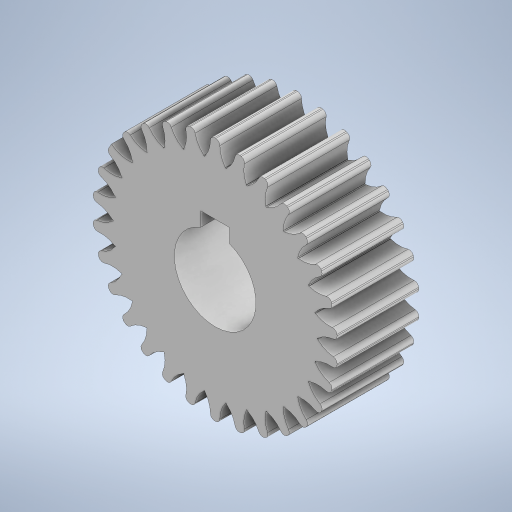
# Autodesk Inventor part: ENGRANE
Saved by Autodesk Inventor 2024 (Build 280153000, 153)
## iProperties
Created: 2024-03-04
Part Number: ENGRANE
Material: Generic
Document SubType Name: Modeling
Designer: augus
Density: 1 g/cm^3
Appearance: Default
Author: augus
Autodesk Inventor part; units mm, degrees
ref_plane "YZ Plane" through (0, 0, 0) normal (1, 0, 0) x (0, 1, 0)
ref_plane "XZ Plane" through (0, 0, 0) normal (0, 1, 0) x (-1, 0, 0)
ref_plane "XY Plane" through (0, 0, 0) normal (0, 0, 1) x (1, 0, 0)
sketch "Sketch1" plane through (0, 0, 0) normal (0, 0, 1) x (1, 0, 0)
  circle A0 centre (0, 0) radius 25
  line L0 (-1.25, 30) -> (1.25, 30)
  line L1 (2.5, 25) -> (2.5, 20)
  line L2 (2.5, 20) -> (-2.5, 20)
  line L3 (-2.5, 20) -> (-2.5, 25)
  line L4 (-1.2964, 27.5929) -> (2.5, 20) construction
  line L5 (1.2964, 27.5929) -> (-2.5, 20) construction
  arc A1 (-2.5, 25) -> (-1.25, 30) centre (-7.5449, 28.9175) ccw
  arc A2 (1.25, 30) -> (2.5, 25) centre (7.5449, 28.9175) ccw
  line L6 (-7.46, 29.0845) -> (-5.0147, 29.6043)
  arc A3 (-5.0147, 29.6043) -> (-2.7524, 24.9735) centre (1.3677, 29.8542) ccw
  arc A4 (-7.6432, 23.9339) -> (-7.46, 29.0845) centre (-13.3923, 26.7169) ccw
  line L7 (-6.6036, 19.0432) -> (-7.6432, 23.9339)
  line L8 (-2.7524, 24.9735) -> (-1.7129, 20.0827)
  line L9 (-1.7129, 20.0827) -> (-6.6036, 19.0432)
  line L10 (-13.344, 26.8979) -> (-11.0602, 27.9148)
  arc A5 (-11.0602, 27.9148) -> (-7.8846, 23.8555) centre (-4.8692, 29.4862) ccw
  arc A6 (-12.4523, 21.8218) -> (-13.344, 26.8979) centre (-18.6544, 23.3486) ccw
  line L11 (-10.4186, 17.2541) -> (-12.4523, 21.8218)
  line L12 (-7.8846, 23.8555) -> (-5.8509, 19.2878)
  line L13 (-5.8509, 19.2878) -> (-10.4186, 17.2541)
  line L14 (-18.6448, 23.5358) -> (-16.6223, 25.0052)
  arc A7 (-16.6223, 25.0052) -> (-12.6721, 21.6949) centre (-10.8933, 27.8295) ccw
  arc A8 (-16.7172, 18.756) -> (-18.6448, 23.5358) centre (-23.1012, 18.96) ccw
  line L15 (-13.7782, 14.7109) -> (-16.7172, 18.756)
  line L16 (-12.6721, 21.6949) -> (-9.7332, 17.6498)
  line L17 (-9.7332, 17.6498) -> (-13.7782, 14.7109)
  line L18 (-23.1308, 19.145) -> (-21.4579, 21.0028)
  arc A9 (-21.4579, 21.0028) -> (-16.9058, 18.5861) centre (-16.4414, 24.9565) ccw
  arc A10 (-20.2514, 14.8704) -> (-23.1308, 19.145) centre (-26.5384, 13.7426) ccw
  line L19 (-16.5357, 11.5248) -> (-20.2514, 14.8704)
  line L20 (-16.9058, 18.5861) -> (-13.1901, 15.2405)
  line L21 (-13.1901, 15.2405) -> (-16.5357, 11.5248)
  line L22 (-26.6058, 13.9175) -> (-25.3558, 16.0825)
  arc A11 (-25.3558, 16.0825) -> (-20.4006, 14.6651) centre (-21.2708, 20.9928) ccw
  arc A12 (-22.9006, 10.3349) -> (-26.6058, 13.9175) centre (-28.8157, 7.9247) ccw
  line L23 (-18.5705, 7.8349) -> (-22.9006, 10.3349)
  line L24 (-20.4006, 14.6651) -> (-16.0705, 12.1651)
  line L25 (-16.0705, 12.1651) -> (-18.5705, 7.8349)
  line L26 (-28.918, 8.0817) -> (-28.1454, 10.4593)
  arc A13 (-28.1454, 10.4593) -> (-23.0039, 10.1031) centre (-25.1707, 16.1116) ccw
  arc A14 (-24.549, 5.3478) -> (-28.918, 8.0817) centre (-29.8336, 1.7604) ccw
  line L27 (-19.7937, 3.8027) -> (-24.549, 5.3478)
  line L28 (-23.0039, 10.1031) -> (-18.2486, 8.558)
  line L29 (-18.2486, 8.558) -> (-19.7937, 3.8027)
  line L30 (-29.9663, 1.8927) -> (-29.705, 4.379)
  arc A15 (-29.705, 4.379) -> (-24.6017, 5.0995) centre (-27.9704, 10.5262) ccw
  arc A16 (-25.1244, 0.1269) -> (-29.9663, 1.8927) centre (-29.5477, -4.4808) ccw
  line L31 (-20.1518, -0.3957) -> (-25.1244, 0.1269)
  line L32 (-24.6017, 5.0995) -> (-19.6291, 4.5769)
  line L33 (-19.6291, 4.5769) -> (-20.1518, -0.3957)
  line L34 (-29.705, -4.379) -> (-29.9663, -1.8927)
  arc A17 (-29.9663, -1.8927) -> (-25.1244, -0.1269) centre (-29.5477, 4.4808) ccw
  arc A18 (-24.6017, -5.0995) -> (-29.705, -4.379) centre (-27.9704, -10.5262) ccw
  line L35 (-19.6291, -4.5769) -> (-24.6017, -5.0995)
  line L36 (-25.1244, -0.1269) -> (-20.1518, 0.3957)
  line L37 (-20.1518, 0.3957) -> (-19.6291, -4.5769)
  line L38 (-28.1454, -10.4593) -> (-28.918, -8.0817)
  arc A19 (-28.918, -8.0817) -> (-24.549, -5.3478) centre (-29.8336, -1.7604) ccw
  arc A20 (-23.0039, -10.1031) -> (-28.1454, -10.4593) centre (-25.1707, -16.1116) ccw
  line L39 (-18.2486, -8.558) -> (-23.0039, -10.1031)
  line L40 (-24.549, -5.3478) -> (-19.7937, -3.8027)
  line L41 (-19.7937, -3.8027) -> (-18.2486, -8.558)
  line L42 (-25.3558, -16.0825) -> (-26.6058, -13.9175)
  arc A21 (-26.6058, -13.9175) -> (-22.9006, -10.3349) centre (-28.8157, -7.9247) ccw
  arc A22 (-20.4006, -14.6651) -> (-25.3558, -16.0825) centre (-21.2708, -20.9928) ccw
  line L43 (-16.0705, -12.1651) -> (-20.4006, -14.6651)
  line L44 (-22.9006, -10.3349) -> (-18.5705, -7.8349)
  line L45 (-18.5705, -7.8349) -> (-16.0705, -12.1651)
  line L46 (-21.4579, -21.0028) -> (-23.1308, -19.145)
  arc A23 (-23.1308, -19.145) -> (-20.2514, -14.8704) centre (-26.5384, -13.7426) ccw
  arc A24 (-16.9058, -18.5861) -> (-21.4579, -21.0028) centre (-16.4414, -24.9565) ccw
  line L47 (-13.1901, -15.2405) -> (-16.9058, -18.5861)
  line L48 (-20.2514, -14.8704) -> (-16.5357, -11.5248)
  line L49 (-16.5357, -11.5248) -> (-13.1901, -15.2405)
  line L50 (-16.6223, -25.0052) -> (-18.6448, -23.5358)
  arc A25 (-18.6448, -23.5358) -> (-16.7172, -18.756) centre (-23.1012, -18.96) ccw
  arc A26 (-12.6721, -21.6949) -> (-16.6223, -25.0052) centre (-10.8933, -27.8295) ccw
  line L51 (-9.7332, -17.6498) -> (-12.6721, -21.6949)
  line L52 (-16.7172, -18.756) -> (-13.7782, -14.7109)
  line L53 (-13.7782, -14.7109) -> (-9.7332, -17.6498)
  line L54 (-11.0602, -27.9148) -> (-13.344, -26.8979)
  arc A27 (-13.344, -26.8979) -> (-12.4523, -21.8218) centre (-18.6544, -23.3486) ccw
  arc A28 (-7.8846, -23.8555) -> (-11.0602, -27.9148) centre (-4.8692, -29.4862) ccw
  line L55 (-5.8509, -19.2878) -> (-7.8846, -23.8555)
  line L56 (-12.4523, -21.8218) -> (-10.4186, -17.2541)
  line L57 (-10.4186, -17.2541) -> (-5.8509, -19.2878)
  line L58 (-5.0147, -29.6043) -> (-7.46, -29.0845)
  arc A29 (-7.46, -29.0845) -> (-7.6432, -23.9339) centre (-13.3923, -26.7169) ccw
  arc A30 (-2.7524, -24.9735) -> (-5.0147, -29.6043) centre (1.3677, -29.8542) ccw
  line L59 (-1.7129, -20.0827) -> (-2.7524, -24.9735)
  line L60 (-7.6432, -23.9339) -> (-6.6036, -19.0432)
  line L61 (-6.6036, -19.0432) -> (-1.7129, -20.0827)
  line L62 (1.25, -30) -> (-1.25, -30)
  arc A31 (-1.25, -30) -> (-2.5, -25) centre (-7.5449, -28.9175) ccw
  arc A32 (2.5, -25) -> (1.25, -30) centre (7.5449, -28.9175) ccw
  line L63 (2.5, -20) -> (2.5, -25)
  line L64 (-2.5, -25) -> (-2.5, -20)
  line L65 (-2.5, -20) -> (2.5, -20)
  line L66 (7.46, -29.0845) -> (5.0147, -29.6043)
  arc A33 (5.0147, -29.6043) -> (2.7524, -24.9735) centre (-1.3677, -29.8542) ccw
  arc A34 (7.6432, -23.9339) -> (7.46, -29.0845) centre (13.3923, -26.7169) ccw
  line L67 (6.6036, -19.0432) -> (7.6432, -23.9339)
  line L68 (2.7524, -24.9735) -> (1.7129, -20.0827)
  line L69 (1.7129, -20.0827) -> (6.6036, -19.0432)
  line L70 (13.344, -26.8979) -> (11.0602, -27.9148)
  arc A35 (11.0602, -27.9148) -> (7.8846, -23.8555) centre (4.8692, -29.4862) ccw
  arc A36 (12.4523, -21.8218) -> (13.344, -26.8979) centre (18.6544, -23.3486) ccw
  line L71 (10.4186, -17.2541) -> (12.4523, -21.8218)
  line L72 (7.8846, -23.8555) -> (5.8509, -19.2878)
  line L73 (5.8509, -19.2878) -> (10.4186, -17.2541)
  line L74 (18.6448, -23.5358) -> (16.6223, -25.0052)
  arc A37 (16.6223, -25.0052) -> (12.6721, -21.6949) centre (10.8933, -27.8295) ccw
  arc A38 (16.7172, -18.756) -> (18.6448, -23.5358) centre (23.1012, -18.96) ccw
  line L75 (13.7782, -14.7109) -> (16.7172, -18.756)
  line L76 (12.6721, -21.6949) -> (9.7332, -17.6498)
  line L77 (9.7332, -17.6498) -> (13.7782, -14.7109)
  line L78 (23.1308, -19.145) -> (21.4579, -21.0028)
  arc A39 (21.4579, -21.0028) -> (16.9058, -18.5861) centre (16.4414, -24.9565) ccw
  arc A40 (20.2514, -14.8704) -> (23.1308, -19.145) centre (26.5384, -13.7426) ccw
  line L79 (16.5357, -11.5248) -> (20.2514, -14.8704)
  line L80 (16.9058, -18.5861) -> (13.1901, -15.2405)
  line L81 (13.1901, -15.2405) -> (16.5357, -11.5248)
  line L82 (26.6058, -13.9175) -> (25.3558, -16.0825)
  arc A41 (25.3558, -16.0825) -> (20.4006, -14.6651) centre (21.2708, -20.9928) ccw
  arc A42 (22.9006, -10.3349) -> (26.6058, -13.9175) centre (28.8157, -7.9247) ccw
  line L83 (18.5705, -7.8349) -> (22.9006, -10.3349)
  line L84 (20.4006, -14.6651) -> (16.0705, -12.1651)
  line L85 (16.0705, -12.1651) -> (18.5705, -7.8349)
  line L86 (28.918, -8.0817) -> (28.1454, -10.4593)
  arc A43 (28.1454, -10.4593) -> (23.0039, -10.1031) centre (25.1707, -16.1116) ccw
  arc A44 (24.549, -5.3478) -> (28.918, -8.0817) centre (29.8336, -1.7604) ccw
  line L87 (19.7937, -3.8027) -> (24.549, -5.3478)
  line L88 (23.0039, -10.1031) -> (18.2486, -8.558)
  line L89 (18.2486, -8.558) -> (19.7937, -3.8027)
  line L90 (29.9663, -1.8927) -> (29.705, -4.379)
  arc A45 (29.705, -4.379) -> (24.6017, -5.0995) centre (27.9704, -10.5262) ccw
  arc A46 (25.1244, -0.1269) -> (29.9663, -1.8927) centre (29.5477, 4.4808) ccw
  line L91 (20.1518, 0.3957) -> (25.1244, -0.1269)
  line L92 (24.6017, -5.0995) -> (19.6291, -4.5769)
  line L93 (19.6291, -4.5769) -> (20.1518, 0.3957)
  line L94 (29.705, 4.379) -> (29.9663, 1.8927)
  arc A47 (29.9663, 1.8927) -> (25.1244, 0.1269) centre (29.5477, -4.4808) ccw
  arc A48 (24.6017, 5.0995) -> (29.705, 4.379) centre (27.9704, 10.5262) ccw
  line L95 (19.6291, 4.5769) -> (24.6017, 5.0995)
  line L96 (25.1244, 0.1269) -> (20.1518, -0.3957)
  line L97 (20.1518, -0.3957) -> (19.6291, 4.5769)
  line L98 (28.1454, 10.4593) -> (28.918, 8.0817)
  arc A49 (28.918, 8.0817) -> (24.549, 5.3478) centre (29.8336, 1.7604) ccw
  arc A50 (23.0039, 10.1031) -> (28.1454, 10.4593) centre (25.1707, 16.1116) ccw
  line L99 (18.2486, 8.558) -> (23.0039, 10.1031)
  line L100 (24.549, 5.3478) -> (19.7937, 3.8027)
  line L101 (19.7937, 3.8027) -> (18.2486, 8.558)
  line L102 (25.3558, 16.0825) -> (26.6058, 13.9175)
  arc A51 (26.6058, 13.9175) -> (22.9006, 10.3349) centre (28.8157, 7.9247) ccw
  arc A52 (20.4006, 14.6651) -> (25.3558, 16.0825) centre (21.2708, 20.9928) ccw
  line L103 (16.0705, 12.1651) -> (20.4006, 14.6651)
  line L104 (22.9006, 10.3349) -> (18.5705, 7.8349)
  line L105 (18.5705, 7.8349) -> (16.0705, 12.1651)
  line L106 (21.4579, 21.0028) -> (23.1308, 19.145)
  arc A53 (23.1308, 19.145) -> (20.2514, 14.8704) centre (26.5384, 13.7426) ccw
  arc A54 (16.9058, 18.5861) -> (21.4579, 21.0028) centre (16.4414, 24.9565) ccw
  line L107 (13.1901, 15.2405) -> (16.9058, 18.5861)
  line L108 (20.2514, 14.8704) -> (16.5357, 11.5248)
  line L109 (16.5357, 11.5248) -> (13.1901, 15.2405)
  line L110 (16.6223, 25.0052) -> (18.6448, 23.5358)
  arc A55 (18.6448, 23.5358) -> (16.7172, 18.756) centre (23.1012, 18.96) ccw
  arc A56 (12.6721, 21.6949) -> (16.6223, 25.0052) centre (10.8933, 27.8295) ccw
  line L111 (9.7332, 17.6498) -> (12.6721, 21.6949)
  line L112 (16.7172, 18.756) -> (13.7782, 14.7109)
  line L113 (13.7782, 14.7109) -> (9.7332, 17.6498)
  line L114 (11.0602, 27.9148) -> (13.344, 26.8979)
  arc A57 (13.344, 26.8979) -> (12.4523, 21.8218) centre (18.6544, 23.3486) ccw
  arc A58 (7.8846, 23.8555) -> (11.0602, 27.9148) centre (4.8692, 29.4862) ccw
  line L115 (5.8509, 19.2878) -> (7.8846, 23.8555)
  line L116 (12.4523, 21.8218) -> (10.4186, 17.2541)
  line L117 (10.4186, 17.2541) -> (5.8509, 19.2878)
  line L118 (5.0147, 29.6043) -> (7.46, 29.0845)
  arc A59 (7.46, 29.0845) -> (7.6432, 23.9339) centre (13.3923, 26.7169) ccw
  arc A60 (2.7524, 24.9735) -> (5.0147, 29.6043) centre (-1.3677, 29.8542) ccw
  line L119 (1.7129, 20.0827) -> (2.7524, 24.9735)
  line L120 (7.6432, 23.9339) -> (6.6036, 19.0432)
  line L121 (6.6036, 19.0432) -> (1.7129, 20.0827)
  point P0 (-7.005, 26.7204)
  point P1 (-4.4688, 27.2595)
  point P2 (-12.4074, 24.6801)
  point P3 (-10.0387, 25.7347)
  point P4 (-17.2675, 21.5611)
  point P5 (-15.1698, 23.0852)
  point P6 (-21.373, 17.4998)
  point P7 (-19.638, 19.4267)
  point P8 (-24.5444, 12.6737)
  point P9 (-23.2479, 14.9192)
  point P10 (-26.643, 7.2937)
  point P11 (-25.8418, 9.7597)
  point P12 (-27.5773, 1.5949)
  point P13 (-27.3062, 4.1736)
  point P14 (-27.3062, -4.1736)
  point P15 (-27.5773, -1.5949)
  point P16 (-25.8418, -9.7597)
  point P17 (-26.643, -7.2937)
  point P18 (-23.2479, -14.9192)
  point P19 (-24.5444, -12.6737)
  point P20 (-19.638, -19.4267)
  point P21 (-21.373, -17.4998)
  point P22 (-15.1698, -23.0852)
  point P23 (-17.2675, -21.5611)
  point P24 (-10.0387, -25.7347)
  point P25 (-12.4074, -24.6801)
  point P26 (-4.4688, -27.2595)
  point P27 (-7.005, -26.7204)
  point P28 (1.2964, -27.5929)
  point P29 (-1.2964, -27.5929)
  point P30 (7.005, -26.7204)
  point P31 (4.4688, -27.2595)
  point P32 (12.4074, -24.6801)
  point P33 (10.0387, -25.7347)
  point P34 (17.2675, -21.5611)
  point P35 (15.1698, -23.0852)
  point P36 (21.373, -17.4998)
  point P37 (19.638, -19.4267)
  point P38 (24.5444, -12.6737)
  point P39 (23.2479, -14.9192)
  point P40 (26.643, -7.2937)
  point P41 (25.8418, -9.7597)
  point P42 (27.5773, -1.5949)
  point P43 (27.3062, -4.1736)
  point P44 (27.3062, 4.1736)
  point P45 (27.5773, 1.5949)
  point P46 (25.8418, 9.7597)
  point P47 (26.643, 7.2937)
  point P48 (23.2479, 14.9192)
  point P49 (24.5444, 12.6737)
  point P50 (19.638, 19.4267)
  point P51 (21.373, 17.4998)
  point P52 (15.1698, 23.0852)
  point P53 (17.2675, 21.5611)
  point P54 (10.0387, 25.7347)
  point P55 (12.4074, 24.6801)
  point P56 (4.4688, 27.2595)
  point P57 (7.005, 26.7204)
  point P58 (-2.5, 24.8747)
  point P59 (-2.7264, 24.8509)
  point P60 (-7.6171, 23.8113)
  point P61 (-7.8336, 23.741)
  point P62 (-12.4013, 21.7073)
  point P63 (-12.5984, 21.5935)
  point P64 (-16.6435, 18.6546)
  point P65 (-16.8127, 18.5023)
  point P66 (-20.1583, 14.7866)
  point P67 (-20.2921, 14.6024)
  point P68 (-22.7921, 10.2723)
  point P69 (-22.8847, 10.0643)
  point P70 (-24.4298, 5.3091)
  point P71 (-24.4771, 5.0864)
  point P72 (-24.9997, 0.1138)
  point P73 (-24.9997, -0.1138)
  point P74 (-24.4771, -5.0864)
  point P75 (-24.4298, -5.3091)
  point P76 (-22.8847, -10.0643)
  point P77 (-22.7921, -10.2723)
  point P78 (-20.2921, -14.6024)
  point P79 (-20.1583, -14.7866)
  point P80 (-16.8127, -18.5023)
  point P81 (-16.6435, -18.6546)
  point P82 (-12.5984, -21.5935)
  point P83 (-12.4013, -21.7073)
  point P84 (-7.8336, -23.741)
  point P85 (-7.6171, -23.8113)
  point P86 (-2.7264, -24.8509)
  point P87 (-2.5, -24.8747)
  point P88 (2.5, -24.8747)
  point P89 (2.7264, -24.8509)
  point P90 (7.6171, -23.8113)
  point P91 (7.8336, -23.741)
  point P92 (12.4013, -21.7073)
  point P93 (12.5984, -21.5935)
  point P94 (16.6435, -18.6546)
  point P95 (16.8127, -18.5023)
  point P96 (20.1583, -14.7866)
  point P97 (20.2921, -14.6024)
  point P98 (22.7921, -10.2723)
  point P99 (22.8847, -10.0643)
  point P100 (24.4298, -5.3091)
  point P101 (24.4771, -5.0864)
  point P102 (24.9997, -0.1138)
  point P103 (24.9997, 0.1138)
  point P104 (24.4771, 5.0864)
  point P105 (24.4298, 5.3091)
  point P106 (22.8847, 10.0643)
  point P107 (22.7921, 10.2723)
  point P108 (20.2921, 14.6024)
  point P109 (20.1583, 14.7866)
  point P110 (16.8127, 18.5023)
  point P111 (16.6435, 18.6546)
  point P112 (12.5984, 21.5935)
  point P113 (12.4013, 21.7073)
  point P114 (7.8336, 23.741)
  point P115 (7.6171, 23.8113)
  point P116 (2.7264, 24.8509)
  point P117 (2.5, 24.8747)
  dimension "d0" = 50
  dimension "d1" = 5
  dimension "d5" = 360
  constraints: 244 end point, 180 point on circle, 60 centre point, 2 parallel, 1 coincident, 1 horizontal, 1 perpendicular, 483 other
  measures "d1" distance of L1.end L2.end
extrude "Extrusion1" add sketch "Sketch1" along normal blind 20
fillet "Fillet1" radius 1 59 edges at (-13.344, 26.8979, 10) (-11.0602, 27.9148, 10) (-7.46, 29.0845, 10) (-5.0147, 29.6043, 10) (-1.25, 30, 10) (1.25, 30, 10) (5.0147, 29.6043, 10) (7.46, 29.0845, 10) (11.0602, 27.9148, 10) (13.344, 26.8979, 10) (16.6223, 25.0052, 10) (18.6448, 23.5358, 10) (21.4579, 21.0028, 10) (23.1308, 19.145, 10) (25.3558, 16.0825, 10) (26.6058, 13.9175, 10) (28.1454, 10.4593, 10) (28.918, 8.0817, 10) (29.705, 4.379, 10) (29.9663, 1.8927, 10) (29.9663, -1.8927, 10) (29.705, -4.379, 10) (28.918, -8.0817, 10) (28.1454, -10.4593, 10) (26.6058, -13.9175, 10) (25.3558, -16.0825, 10) (23.1308, -19.145, 10) (21.4579, -21.0028, 10) (18.6448, -23.5358, 10) (16.6223, -25.0052, 10) (13.344, -26.8979, 10) (11.0602, -27.9148, 10) (7.46, -29.0845, 10) (5.0147, -29.6043, 10) (1.25, -30, 10) (-1.25, -30, 10) (-5.0147, -29.6043, 10) (-7.46, -29.0845, 10) (-11.0602, -27.9148, 10) (-13.344, -26.8979, 10) (-16.6223, -25.0052, 10) (-18.6448, -23.5358, 10) (-21.4579, -21.0028, 10) (-23.1308, -19.145, 10) (-25.3558, -16.0825, 10) (-26.6058, -13.9175, 10) (-28.1454, -10.4593, 10) (-28.918, -8.0817, 10) (-26.6058, 13.9175, 10) (-28.1454, 10.4593, 10) (-28.918, 8.0817, 10) (-29.705, 4.379, 10) (-29.9663, 1.8927, 10) (-29.9663, -1.8927, 10) (-29.705, -4.379, 10) (-23.1308, 19.145, 10) (-21.4579, 21.0028, 10) (-18.6448, 23.5358, 10) (-16.6223, 25.0052, 10)
sketch "Sketch2" plane through (0, 0, 20) normal (0, 0, 1) x (1, 0, 0)
  circle A0 centre (0, 0) radius 10
  dimension "d10" = 20
  constraints: 1 centre point, 1 coincident
  measures "d10" diameter of A0
extrude "Extrusion2" cut sketch "Sketch2" against normal through all
sketch "Sketch3" plane through (0, 0, 20) normal (0, 0, 1) x (1, 0, 0)
  line L0 (-3.5, 7.185) -> (3.5, 7.185)
  line L1 (3.5, 7.185) -> (3.5, 12.815)
  line L2 (3.5, 12.815) -> (-3.5, 12.815)
  line L3 (-3.5, 12.815) -> (-3.5, 7.185)
  circle A0 centre (0, 0) radius 10 projected
  line L4 (-3.5, 7.185) -> (3.5, 12.815) construction
  line L5 (3.5, 7.185) -> (-3.5, 12.815) construction
  point P0 (0, 10)
  dimension "d17" = 7
  dimension "d18" = 5.63
  constraints: 12 end point, 2 midpoint, 2 parallel, 1 horizontal, 1 perpendicular, 1 vertical alignment, 1 other
  measures "d17" distance of L2.end L1.end
  measures "d18" distance of L1.end L0.end
extrude "Extrusion3" cut sketch "Sketch3" against normal through all contours L3 A0 L1 L0 | L3 L2 L1 A0 picked at (0.3964, 8.0997)
body "Solid1"
